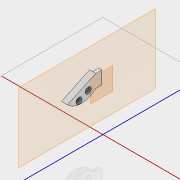
# Autodesk Inventor part: ЛЦМК.30000.10.00.04  Переходник
Saved by Autodesk Inventor 2021.2 (Build 252289000, 289)
## iProperties
Created: 2025-11-22
Part Number: ЛЦМК.30000.10.00.04  Переходник
Material: Типовые
Document SubType Name: Modeling
Designer: Захаров
Density: 1 g/cm^3
Appearance: По умолчанию
Author: Захаров
Autodesk Inventor part; units mm, degrees
ref_plane "YZ Plane" through (0, 0, 0) normal (1, 0, 0) x (0, 1, 0)
ref_plane "XZ Plane" through (0, 0, 0) normal (0, 1, 0) x (-1, 0, 0)
ref_plane "XY Plane" through (0, 0, 0) normal (0, 0, 1) x (1, 0, 0)
sketch "Эскиз1" plane through (0, 0, 0) normal (0, 0, 1) x (1, 0, 0)
  line L0 (-10, 17) -> (-7, 17) projected
  line L1 (-10, 4) -> (-10, 17) projected
  line L2 (-7, 4) -> (-10, 4) projected
  line L3 (-7, 17) -> (-7, 4) projected
  line L4 (-9.9, 4.1) -> (-9.9, 16.9)
  line L5 (-9.9, 16.9) -> (-7.1, 16.9)
  line L6 (-7.1, 16.9) -> (-7.1, 4.1)
  line L7 (-7.1, 4.1) -> (-9.9, 4.1)
  point P0 (0, 0)
  dimension "d22" = 0.1
  constraints: 8 end point, 3 other
  measures "d22" distance between parallel lines of L2 L7
ref_plane "РабПлоскость1" through (-13, -24, -6) normal (0, 0, -1) x (0, 1, 0)
extrude "Выдавливание1" add sketch "Эскиз1" against normal up to surface (6 mm away) contours L4 L5 L6 L7
ref_plane "РабПлоскость2" through (-13, 2.5481, 2.5558) normal (1, 0, 0) x (0, 1, 0)
sketch "Эскиз3" plane through (-13, 2.5481, 2.5558) normal (1, 0, 0) x (0, 1, 0)
  line L0 (29.663, -39.7893) -> (-15.8657, 56.6115) projected
  line L1 (1.4519, -2.5558) -> (14.4519, -2.5558) projected
  circle A0 centre (3.4507, 4.8159) radius 1.5 projected
  circle A1 centre (-0.8198, 13.8581) radius 1.5 projected
  arc A2 (1.3781, 25.1262) -> (1.4519, -2.5558) centre (15.5518, 11.3229) ccw
  line L2 (31.6038, -38.8726) -> (-13.9249, 57.5281)
  point P0 (-2.5481, -2.5558)
  point P1 (-0.157, 23.3504)
  point P2 (12.0781, -2.5558)
  constraints: 3 point on circle, 2 end point, 2 point on line, 1 centre point, 1 parallel
ref_plane "РабПлоскость3" through (-7, 4, -6) normal (-1, 0, 0) x (0, 0, 1)
extrude "Выдавливание3" add sketch "Эскиз3" along normal up to surface (6 mm away)
ref_plane "РабПлоскость5" through (-7, 4.2958, -6) normal (1, 0, 0) x (0, 0, -1)
sketch "Эскиз5" plane through (-7, 4.2958, -6) normal (1, 0, 0) x (0, 0, -1)
  spline S0 degree 2 poles (-13.3717, 3.2031) (-15.9697, 3.2031) (-14.6707, 0.9531) (-13.3717, -1.2969) (-12.0726, 0.9531) (-10.7736, 3.2031) (-13.3717, 3.2031) knots 0 0 0 0.333333 0.333333 0.666667 0.666667 1 1 1 weights 1 0.5 1 0.5 1 0.5 1 projected
  circle A0 centre (-13.3717, 1.7031) radius 3
  circle A1 centre (-13.3717, 1.7031) radius 1.5 projected
  circle A2 centre (-13.3717, 1.7031) radius 1.5 projected
  point P0 (-6, -4.2958)
  point P1 (-23.7703, -3.2081)
  point P2 (-23.7703, -3.2081)
  dimension "d12" = 6
  constraints: 1 centre point, 1 concentric, 1 other
  measures "d12" diameter of A0
extrude "Выдавливание5" cut sketch "Эскиз5" against normal blind 2.5
ref_plane "РабПлоскость4" through (-7, 4.2958, -6) normal (1, 0, 0) x (0, 0, -1)
sketch "Эскиз6" plane through (-7, 4.2958, -6) normal (1, 0, 0) x (0, 0, -1)
  spline S0 degree 2 poles (-22.4139, -1.0675) (-25.012, -1.0675) (-23.713, -3.3175) (-22.4139, -5.5675) (-21.1149, -3.3175) (-19.8159, -1.0675) (-22.4139, -1.0675) knots 0 0 0 0.333333 0.333333 0.666667 0.666667 1 1 1 weights 1 0.5 1 0.5 1 0.5 1 projected
  circle A0 centre (-22.4139, -2.5675) radius 1.5 projected
  circle A1 centre (-22.4139, -2.5675) radius 3
  point P0 (-6, -4.2958)
  dimension "d16" = 6
  constraints: 1 centre point, 1 coincident, 2 other
  measures "d16" diameter of A1
extrude "Выдавливание6" cut sketch "Эскиз6" against normal blind 4
sketch "Эскиз7" plane through (-7.1, 4, -6) normal (1, 0, 0) x (0, 0, -1)
  line L0 (-6, 13) -> (0, 13) projected
  line L1 (-6, 13) -> (-33.682, -0.0738) projected
  line L2 (-33.682, -0.0738) -> (-11.0375, 13)
  line L3 (-6, 13) -> (0, 13) projected
  line L4 (-6, 13) -> (-11.0375, 13)
  point P0 (-6, -4)
  dimension "d19" = 30
  constraints: 4 end point, 1 collinear, 1 point on line
  measures "d19" angle of L0 L2
ref_plane "РабПлоскость6" through (-13, -28.5514, -58.6393) normal (1, 0, 0) x (0, 1, 0)
extrude "Выдавливание7" add sketch "Эскиз7" against normal up to surface (5.9 mm away)
